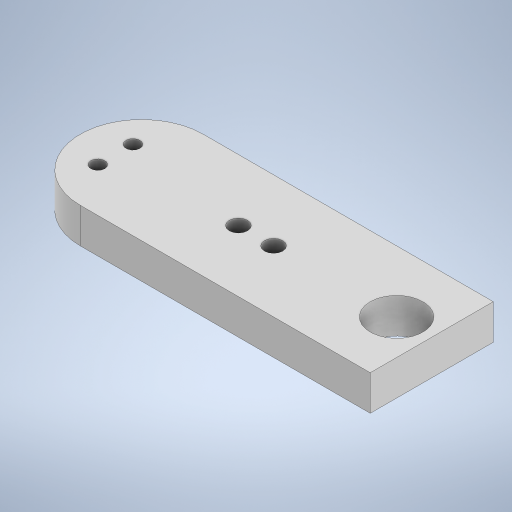
# Autodesk Inventor part: 다리-2
Saved by Autodesk Inventor 2024 (Build 280153000, 153)
## iProperties
Created: 2024-09-10
Part Number: 다리-2
Material: 일반
Document SubType Name: Modeling
Designer: USER
Density: 1 g/cm^3
Appearance: 기본값
Author: USER
Autodesk Inventor part; units mm, degrees
sketch "스케치1" plane through (0, 0, 0) normal (0, 0, 1) x (1, 0, 0)
  line L0 (0, 0) -> (100, 0)
  line L1 (100, 0) -> (100, 10)
  line L2 (100, 10) -> (0, 10)
  line L3 (0, 10) -> (0, 0)
  dimension "d0" = 100
  dimension "d1" = 10
  constraints: 8 end point, 2 parallel, 1 horizontal, 1 perpendicular
  measures "d0" distance of L1.end L2.end
  measures "d1" distance between parallel lines of L0 L2
extrude "돌출1" add sketch "스케치1" along normal blind 35
sketch "스케치3" plane through (0, 0, 0) normal (0, -1, 0) x (1, 0, 0)
  line L0 (0, 0) -> (100, 0) projected
  line L1 (100, 0) -> (100, 35) projected
  line L2 (0, 35) -> (100, 35) projected
  line L3 (0, 0) -> (0, 35) projected
  circle A0 centre (90, 17.5) radius 7.5
  point P0 (15, 17.5)
  point P1 (100, 17.5)
  dimension "d8" = 15
  dimension "d12" = 10
  constraints: 2 horizontal alignment, 1 centre point, 1 midpoint
  measures "d8" diameter of A0
  measures "d12" distance from line of L1 A0.centre
extrude "돌출3" cut sketch "스케치3" against normal through all contours A0
ref_plane "작업 평면1" through (50, 0, 0) normal (-1, 0, 0) x (0, 0, 1)
ref_plane "작업 평면2" through (65, 40, 45) normal (0, 1, 0) x (1, 0, 0)
ref_plane "작업 평면3" through (50, 0, 0) normal (1, 0, 0) x (0, 0, -1)
sketch "스케치4" plane through (0, 10, 0) normal (0, 1, 0) x (1, 0, 0)
  circle A0 centre (90, -17.5) radius 7.5 projected
  line L0 (100, 0) -> (0, 0) projected
  line L1 (0, 0) -> (0, -35) projected
  line L2 (100, -35) -> (0, -35) projected
  line L3 (100, 0) -> (100, -35) projected
  circle A1 centre (45, -17.5) radius 2.6
  circle A2 centre (55, -17.5) radius 2.6
  line L4 (100, 0) -> (0, 0) projected
  point P0 (50, 0)
  point P1 (50, 0)
  point P2 (100, -17.5)
  dimension "d16" = 5.2
  dimension "d17" = 5.2
  dimension "d18" = 10
  dimension "d19" = 5
  constraints: 3 midpoint, 2 centre point, 2 horizontal alignment
  measures "d16" diameter of A2
  measures "d17" diameter of A1
  measures "d18" distance of A2.centre A1.centre
  measures "d19" horizontal distance of A1.centre point (50, 0)
extrude "돌출4" cut sketch "스케치4" against normal through all contours A1 | A2
sketch "스케치5" plane through (0, 10, 0) normal (0, 1, 0) x (1, 0, 0)
  circle A0 centre (10, -12.5) radius 2
  circle A1 centre (10, -22.5) radius 2
  line L0 (0, 0) -> (0, -35) projected
  point P0 (0, -17.5)
  dimension "d20" = 4
  dimension "d21" = 4
  dimension "d22" = 10
  dimension "d23" = 5
  dimension "d24" = 10
  constraints: 2 centre point, 1 midpoint, 1 vertical alignment
  measures "d20" diameter of A0
  measures "d21" diameter of A1
  measures "d22" distance of A0.centre A1.centre
  measures "d23" vertical distance of point (0, -17.5) A0.centre
  measures "d24" distance from line of L0 A0.centre
extrude "돌출5" cut sketch "스케치5" against normal through all
fillet "모깎기1" radius 17.5 2 edges at (0, 5, 0) (0, 5, 35)
